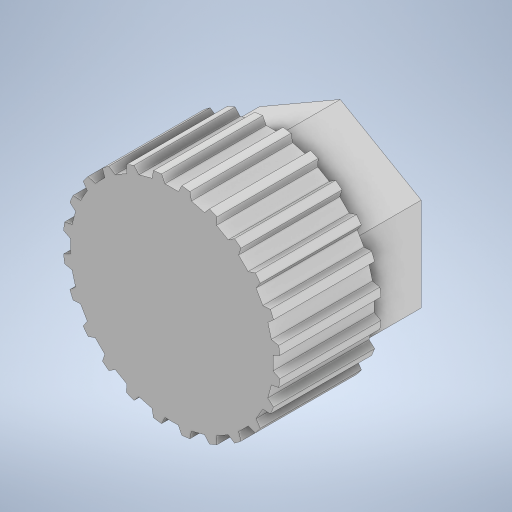
# Autodesk Inventor part: Nastavek Millard freewheel tool izmerjen trapze
Saved by Autodesk Inventor 2023.3 (Build 273359000, 359)
## iProperties
Created: 2024-05-29
Part Number: Nastavek Millard freewheel tool izmerjen trapze
Material: Generic
Document SubType Name: Modeling
Designer: David Zindović
Density: 1 g/cm^3
Appearance: Default
Author: David Zindović
Autodesk Inventor part; units mm, degrees
ref_plane "YZ Plane" through (0, 0, 0) normal (1, 0, 0) x (0, 1, 0)
ref_plane "XZ Plane" through (0, 0, 0) normal (0, 1, 0) x (-1, 0, 0)
ref_plane "XY Plane" through (0, 0, 0) normal (0, 0, 1) x (1, 0, 0)
sketch "Sketch1" plane through (0, 0, 0) normal (0, 0, 1) x (1, 0, 0)
  circle A0 centre (0, 0) radius 17.25
  circle A1 centre (0, 0) radius 16.1
  circle A2 centre (0, 0) radius 15
  line L0 (-1, -15.03) -> (1, -15.03)
  line L1 (-1.5, -16.03) -> (1.5, -16.03)
  line L2 (1.5, -16.03) -> (1, -15.03)
  line L3 (-1.5, -16.03) -> (-1, -15.03)
  line L4 (-1, -15.03) -> (-0.9693, -14.9686)
  line L5 (1, -15.03) -> (0.9693, -14.9686)
  line L6 (2.9241, -14.7767) -> (4.856, -14.259)
  line L7 (2.7, -15.872) -> (2.9241, -14.7767)
  line L8 (2.9241, -14.7767) -> (2.9379, -14.7095)
  line L9 (5.5978, -15.0955) -> (4.856, -14.259)
  line L10 (4.856, -14.259) -> (4.8105, -14.2077)
  line L11 (6.649, -13.5163) -> (8.381, -12.5163)
  line L12 (6.7159, -14.6324) -> (6.649, -13.5163)
  line L13 (6.649, -13.5163) -> (6.6449, -13.4479)
  line L14 (9.314, -13.1324) -> (8.381, -12.5163)
  line L15 (8.381, -12.5163) -> (8.3238, -12.4786)
  line L16 (9.9207, -11.3349) -> (11.3349, -9.9207)
  line L17 (10.2742, -12.3956) -> (9.9207, -11.3349)
  line L18 (9.9207, -11.3349) -> (9.899, -11.2699)
  line L19 (12.3956, -10.2742) -> (11.3349, -9.9207)
  line L20 (11.3349, -9.9207) -> (11.2699, -9.899)
  line L21 (12.5163, -8.381) -> (13.5163, -6.649)
  line L22 (13.1324, -9.314) -> (12.5163, -8.381)
  line L23 (12.5163, -8.381) -> (12.4786, -8.3238)
  line L24 (14.6324, -6.7159) -> (13.5163, -6.649)
  line L25 (13.5163, -6.649) -> (13.4479, -6.6449)
  line L26 (14.259, -4.856) -> (14.7767, -2.9241)
  line L27 (15.0955, -5.5978) -> (14.259, -4.856)
  line L28 (14.259, -4.856) -> (14.2077, -4.8105)
  line L29 (15.872, -2.7) -> (14.7767, -2.9241)
  line L30 (14.7767, -2.9241) -> (14.7095, -2.9379)
  line L31 (15.03, -1) -> (15.03, 1)
  line L32 (16.03, -1.5) -> (15.03, -1)
  line L33 (15.03, -1) -> (14.9686, -0.9693)
  line L34 (16.03, 1.5) -> (15.03, 1)
  line L35 (15.03, 1) -> (14.9686, 0.9693)
  line L36 (14.7767, 2.9241) -> (14.259, 4.856)
  line L37 (15.872, 2.7) -> (14.7767, 2.9241)
  line L38 (14.7767, 2.9241) -> (14.7095, 2.9379)
  line L39 (15.0955, 5.5978) -> (14.259, 4.856)
  line L40 (14.259, 4.856) -> (14.2077, 4.8105)
  line L41 (13.5163, 6.649) -> (12.5163, 8.381)
  line L42 (14.6324, 6.7159) -> (13.5163, 6.649)
  line L43 (13.5163, 6.649) -> (13.4479, 6.6449)
  line L44 (13.1324, 9.314) -> (12.5163, 8.381)
  line L45 (12.5163, 8.381) -> (12.4786, 8.3238)
  line L46 (11.3349, 9.9207) -> (9.9207, 11.3349)
  line L47 (12.3956, 10.2742) -> (11.3349, 9.9207)
  line L48 (11.3349, 9.9207) -> (11.2699, 9.899)
  line L49 (10.2742, 12.3956) -> (9.9207, 11.3349)
  line L50 (9.9207, 11.3349) -> (9.899, 11.2699)
  line L51 (8.381, 12.5163) -> (6.649, 13.5163)
  line L52 (9.314, 13.1324) -> (8.381, 12.5163)
  line L53 (8.381, 12.5163) -> (8.3238, 12.4786)
  line L54 (6.7159, 14.6324) -> (6.649, 13.5163)
  line L55 (6.649, 13.5163) -> (6.6449, 13.4479)
  line L56 (4.856, 14.259) -> (2.9241, 14.7767)
  line L57 (5.5978, 15.0955) -> (4.856, 14.259)
  line L58 (4.856, 14.259) -> (4.8105, 14.2077)
  line L59 (2.7, 15.872) -> (2.9241, 14.7767)
  line L60 (2.9241, 14.7767) -> (2.9379, 14.7095)
  line L61 (1, 15.03) -> (-1, 15.03)
  line L62 (1.5, 16.03) -> (1, 15.03)
  line L63 (1, 15.03) -> (0.9693, 14.9686)
  line L64 (-1.5, 16.03) -> (-1, 15.03)
  line L65 (-1, 15.03) -> (-0.9693, 14.9686)
  line L66 (-2.9241, 14.7767) -> (-4.856, 14.259)
  line L67 (-2.7, 15.872) -> (-2.9241, 14.7767)
  line L68 (-2.9241, 14.7767) -> (-2.9379, 14.7095)
  line L69 (-5.5978, 15.0955) -> (-4.856, 14.259)
  line L70 (-4.856, 14.259) -> (-4.8105, 14.2077)
  line L71 (-6.649, 13.5163) -> (-8.381, 12.5163)
  line L72 (-6.7159, 14.6324) -> (-6.649, 13.5163)
  line L73 (-6.649, 13.5163) -> (-6.6449, 13.4479)
  line L74 (-9.314, 13.1324) -> (-8.381, 12.5163)
  line L75 (-8.381, 12.5163) -> (-8.3238, 12.4786)
  line L76 (-9.9207, 11.3349) -> (-11.3349, 9.9207)
  line L77 (-10.2742, 12.3956) -> (-9.9207, 11.3349)
  line L78 (-9.9207, 11.3349) -> (-9.899, 11.2699)
  line L79 (-12.3956, 10.2742) -> (-11.3349, 9.9207)
  line L80 (-11.3349, 9.9207) -> (-11.2699, 9.899)
  line L81 (-12.5163, 8.381) -> (-13.5163, 6.649)
  line L82 (-13.1324, 9.314) -> (-12.5163, 8.381)
  line L83 (-12.5163, 8.381) -> (-12.4786, 8.3238)
  line L84 (-14.6324, 6.7159) -> (-13.5163, 6.649)
  line L85 (-13.5163, 6.649) -> (-13.4479, 6.6449)
  line L86 (-14.259, 4.856) -> (-14.7767, 2.9241)
  line L87 (-15.0955, 5.5978) -> (-14.259, 4.856)
  line L88 (-14.259, 4.856) -> (-14.2077, 4.8105)
  line L89 (-15.872, 2.7) -> (-14.7767, 2.9241)
  line L90 (-14.7767, 2.9241) -> (-14.7095, 2.9379)
  line L91 (-15.03, 1) -> (-15.03, -1)
  line L92 (-16.03, 1.5) -> (-15.03, 1)
  line L93 (-15.03, 1) -> (-14.9686, 0.9693)
  line L94 (-16.03, -1.5) -> (-15.03, -1)
  line L95 (-15.03, -1) -> (-14.9686, -0.9693)
  line L96 (-14.7767, -2.9241) -> (-14.259, -4.856)
  line L97 (-15.872, -2.7) -> (-14.7767, -2.9241)
  line L98 (-14.7767, -2.9241) -> (-14.7095, -2.9379)
  line L99 (-15.0955, -5.5978) -> (-14.259, -4.856)
  line L100 (-14.259, -4.856) -> (-14.2077, -4.8105)
  line L101 (-13.5163, -6.649) -> (-12.5163, -8.381)
  line L102 (-14.6324, -6.7159) -> (-13.5163, -6.649)
  line L103 (-13.5163, -6.649) -> (-13.4479, -6.6449)
  line L104 (-13.1324, -9.314) -> (-12.5163, -8.381)
  line L105 (-12.5163, -8.381) -> (-12.4786, -8.3238)
  line L106 (-11.3349, -9.9207) -> (-9.9207, -11.3349)
  line L107 (-12.3956, -10.2742) -> (-11.3349, -9.9207)
  line L108 (-11.3349, -9.9207) -> (-11.2699, -9.899)
  line L109 (-10.2742, -12.3956) -> (-9.9207, -11.3349)
  line L110 (-9.9207, -11.3349) -> (-9.899, -11.2699)
  line L111 (-8.381, -12.5163) -> (-6.649, -13.5163)
  line L112 (-9.314, -13.1324) -> (-8.381, -12.5163)
  line L113 (-8.381, -12.5163) -> (-8.3238, -12.4786)
  line L114 (-6.7159, -14.6324) -> (-6.649, -13.5163)
  line L115 (-6.649, -13.5163) -> (-6.6449, -13.4479)
  line L116 (-4.856, -14.259) -> (-2.9241, -14.7767)
  line L117 (-5.5978, -15.0955) -> (-4.856, -14.259)
  line L118 (-4.856, -14.259) -> (-4.8105, -14.2077)
  line L119 (-2.7, -15.872) -> (-2.9241, -14.7767)
  line L120 (-2.9241, -14.7767) -> (-2.9379, -14.7095)
  point P0 (0, -16.03)
  point P1 (0, -15.03)
  point P2 (1.5, -16.03)
  point P3 (1.5, -16.03)
  point P4 (3.89, -14.5178)
  point P5 (7.515, -13.0163)
  point P6 (10.6278, -10.6278)
  point P7 (13.0163, -7.515)
  point P8 (14.5178, -3.89)
  point P9 (15.03, 0)
  point P10 (14.5178, 3.89)
  point P11 (13.0163, 7.515)
  point P12 (10.6278, 10.6278)
  point P13 (7.515, 13.0163)
  point P14 (3.89, 14.5178)
  point P15 (0, 15.03)
  point P16 (-3.89, 14.5178)
  point P17 (-7.515, 13.0163)
  point P18 (-10.6278, 10.6278)
  point P19 (-13.0163, 7.515)
  point P20 (-14.5178, 3.89)
  point P21 (-15.03, 0)
  point P22 (-14.5178, -3.89)
  point P23 (-13.0163, -7.515)
  point P24 (-10.6278, -10.6278)
  point P25 (-7.515, -13.0163)
  point P26 (-3.89, -14.5178)
  point P27 (2.7, -15.872)
  point P28 (5.5978, -15.0955)
  point P29 (6.7159, -14.6324)
  point P30 (9.314, -13.1324)
  point P31 (10.2742, -12.3956)
  point P32 (12.3956, -10.2742)
  point P33 (14.6324, -6.7159)
  point P34 (15.872, -2.7)
  point P35 (16.03, -1.5)
  point P36 (16.03, 1.5)
  point P37 (15.872, 2.7)
  point P38 (15.0955, 5.5978)
  point P39 (14.6324, 6.7159)
  point P40 (13.1324, 9.314)
  point P41 (12.3956, 10.2742)
  point P42 (10.2742, 12.3956)
  point P43 (6.7159, 14.6324)
  point P44 (2.7, 15.872)
  point P45 (1.5, 16.03)
  point P46 (-1.5, 16.03)
  point P47 (-5.5978, 15.0955)
  point P48 (-6.7159, 14.6324)
  point P49 (-10.2742, 12.3956)
  point P50 (-12.3956, 10.2742)
  point P51 (-14.6324, 6.7159)
  point P52 (-15.0955, 5.5978)
  point P53 (-15.872, 2.7)
  point P54 (-16.03, -1.5)
  point P55 (-14.6324, -6.7159)
  point P56 (-12.3956, -10.2742)
  point P57 (-10.2742, -12.3956)
  point P58 (-9.314, -13.1324)
  point P59 (-6.7159, -14.6324)
  point P60 (-5.5978, -15.0955)
  point P61 (-2.7, -15.872)
  dimension "d1" = 32.2
  dimension "d0" = 34.5
  dimension "d2" = 30
  dimension "d3" = 2
  dimension "d4" = 3
  dimension "d5" = 1
  dimension "d20" = 360
  constraints: 242 end point, 3 coincident, 2 centre point, 2 collinear, 2 horizontal, 2 midpoint, 2 point on circle, 2 vertical alignment, 292 other
  measures "d0" diameter of A0
  measures "d2" diameter of A2
  measures "d3" distance of L0.start L0.end
  measures "d4" distance of L1.start L1.end
  measures "d5" distance between parallel lines of L0 L1
extrude "Extrusion1" add sketch "Sketch1" along normal blind 15 contours L34 L35 A2 L38 L37 A1 | A1 L29 L30 A2 L33 L32 | L31 L33 A2 L35 | L39 L40 A2 L43 L42 A1 | L38 A2 L40 L36 | A2 | A1 L24 L25 A2 L28 L27 | L26 L28 A2 L30 | L44 L45 A2 L48 L47 A1 | L43 A2 L45 L41 | A1 L19 L20 A2 L23 L22 | L21 L23 A2 L25 | L49 L50 A2 L53 L52 A1 | L48 A2 L50 L46 | A1 L14 L15 A2 L18 L17 | L16 L18 A2 L20 | L54 L55 A2 L58 L57 A1 | L53 A2 L55 L51 | A1 L9 L10 A2 L13 L12 | L11 L13 A2 L15 | L59 L60 A2 L63 L62 A1 | L58 A2 L60 L56 | A1 L2 L5 A2 L8 L7 | L6 L8 A2 L10 | L64 L65 A2 L68 L67 A1 | L63 A2 L65 L61 | A1 L119 L120 A2 L4 L3 | L69 L70 A2 L73 L72 A1 | L68 A2 L70 L66 | A1 L114 L115 A2 L118 L117 | L116 L118 A2 L120 | L74 L75 A2 L78 L77 A1 | L73 A2 L75 L71 | A1 L109 L110 A2 L113 L112 | L111 L113 A2 L115 | L79 L80 A2 L83 L82 A1 | L78 A2 L80 L76 | A1 L104 L105 A2 L108 L107 | L106 L108 A2 L110 | L84 L85 A2 L88 L87 A1 | L83 A2 L85 L81 | A1 L99 L100 A2 L103 L102 | L101 L103 A2 L105 | L89 L90 A2 L93 L92 A1 | L88 A2 L90 L86 | A1 L94 L95 A2 L98 L97 | L96 L98 A2 L100 | L93 A2 L95 L91
sketch "Sketch2" plane through (0, 0, 0) normal (0, 0, -1) x (-1, 0, 0)
  line L0 (12, 6.9282) -> (12, -6.9282)
  line L1 (12, -6.9282) -> (0, -13.8564)
  line L2 (0, -13.8564) -> (-12, -6.9282)
  line L3 (-12, -6.9282) -> (-12, 6.9282)
  line L4 (-12, 6.9282) -> (0, 13.8564)
  line L5 (0, 13.8564) -> (12, 6.9282)
  point P0 (0, 0)
  point P1 (0, 0)
  dimension "d12" = 24
  constraints: 12 end point, 1 coincident, 1 vertical alignment, 13 other
  measures "d12" distance between parallel lines of L3 L0
extrude "Extrusion2" add sketch "Sketch2" along normal blind 10
sketch "Sketch3" plane through (0, 0, -10) normal (0, 0, -1) x (-1, 0, 0)
  circle A0 centre (0, 0) radius 7.5
  dimension "d15" = 15
  constraints: 1 centre point, 1 coincident
  measures "d15" diameter of A0
extrude "Extrusion3" [suppressed]
sketch "Sketch4" plane through (0, 0, 0) normal (1, 0, 0) x (0, 1, 0)
  line L0 (20.1089, -13.3141) -> (-23.1689, -13.3141)
  line L1 (-23.1689, -13.3141) -> (-23.1689, 5.9253)
  line L2 (-23.1689, 5.9253) -> (20.1089, 5.9253)
  line L3 (20.1089, 5.9253) -> (20.1089, -13.3141)
  point P0 (0, 0)
  constraints: 8 end point, 2 parallel, 1 horizontal, 1 perpendicular
extrude "Extrusion4" [suppressed]
body "Solid1"
